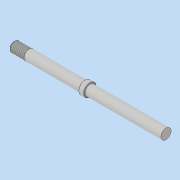
# Autodesk Inventor part: Welle
Saved by Autodesk Inventor 2018 (Build 220112000, 112)
## iProperties
Created: 2020-05-24
Part Number: Welle
Material: Generisch
Document SubType Name: Modeling
Designer: marce
Density: 1 g/cm^3
Appearance: Vorgabe
Author: marce
Autodesk Inventor part; units mm, degrees
ref_plane "YZ Plane" through (0, 0, 0) normal (1, 0, 0) x (0, 1, 0)
ref_plane "XZ Plane" through (0, 0, 0) normal (0, 1, 0) x (-1, 0, 0)
ref_plane "XY Plane" through (0, 0, 0) normal (0, 0, 1) x (1, 0, 0)
sketch "Skizze1" plane through (0, 0, 0) normal (0, 0, 1) x (1, 0, 0)
  line L0 (0, 0) -> (0, 3.95)
  line L1 (0, 3.95) -> (12, 3.95)
  line L2 (12, 3.95) -> (12, 4)
  line L3 (12, 4) -> (56, 4)
  line L4 (56, 4) -> (56, 5)
  line L5 (56, 5) -> (60.1, 5)
  line L6 (60.1, 5) -> (60.1, 4)
  line L7 (60.1, 4) -> (120.1, 4)
  line L8 (120.1, 4) -> (120.1, 0)
  line L9 (120.1, 0) -> (0, 0)
  dimension "d0" = 3.95
  dimension "d1" = 12
  dimension "d3" = 4
  dimension "d6" = 44
  dimension "d8" = 48.1
  dimension "d9" = 5
  dimension "d10" = 60
  constraints: 20 end point, 8 perpendicular, 2 point on line, 1 vertical
  measures "d0" distance between parallel lines of L9 L1
  measures "d1" distance of L0.end L1.end
  measures "d3" distance between parallel lines of L9 L3
  measures "d6" distance between parallel lines of L2 L4
  measures "d8" distance between parallel lines of L2 L6
  measures "d9" distance between parallel lines of L9 L5
  measures "d10" distance of L6.end L7.end
revolve "Umdrehung1" add sketch "Skizze1" angle 360 about axis through (120.1, 0, 0) along (-1, 0, 0)
thread "Gewinde1" size "M8x1.25" class "6g" standard "ANSI Metric M Profile" full length
chamfer "Fase1" distance 0.8 angle 45 1 edges at (0, -3.95, 0)
chamfer "Fase2" distance 0.3 angle 45 2 edges at (56, -5, 0) (60.1, -5, 0)
